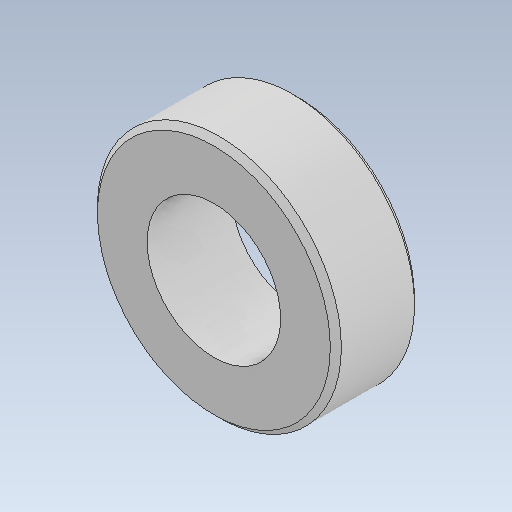
# Autodesk Inventor part: Washer
Saved by Autodesk Inventor 2021 (Build 250183000, 183)
## iProperties
Created: 2022-01-12
Part Number: Washer
Material: Generic
Document SubType Name: Modeling
Designer: stefi
Density: 1 g/cm^3
Appearance: Default
Author: stefi
Autodesk Inventor part; units mm, degrees
ref_plane "YZ Plane" through (0, 0, 0) normal (1, 0, 0) x (0, 1, 0)
ref_plane "XZ Plane" through (0, 0, 0) normal (0, 1, 0) x (-1, 0, 0)
ref_plane "XY Plane" through (0, 0, 0) normal (0, 0, 1) x (1, 0, 0)
sketch "Sketch1" plane through (0, 0, 0) normal (0, 0, 1) x (1, 0, 0)
  circle A0 centre (0, 0) radius 11.03
  circle A1 centre (0, 0) radius 6.035
  dimension "d0" = 22.06
  dimension "d1" = 12.07
  constraints: 2 centre point, 2 coincident
  measures "d0" diameter of A0
  measures "d1" diameter of A1
extrude "Extrusion1" add sketch "Sketch1" along normal blind 7.62
chamfer "Chamfer1" distance 0.5 angle 45 2 edges at (-11.03, 0, 7.62) (-11.03, 0, 0)
body "Solid1"
